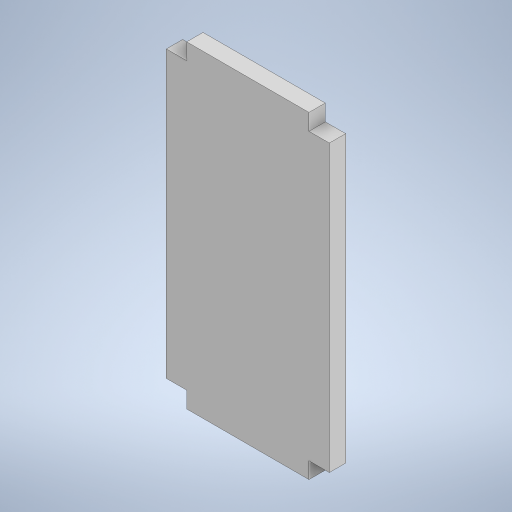
# Autodesk Inventor part: Tussen30_AUG
Saved by Autodesk Inventor 2023.4 (Build 274418000, 418)
## iProperties
Created: 2024-07-29
Part Number: Tussen30_AUG
Material: Generic
Document SubType Name: Modeling
Designer: cthey
Density: 1 g/cm^3
Appearance: Default
Author: cthey
Autodesk Inventor part; units mm, degrees
ref_plane "YZ Plane" through (0, 0, 0) normal (1, 0, 0) x (0, 1, 0)
ref_plane "XZ Plane" through (0, 0, 0) normal (0, 1, 0) x (-1, 0, 0)
ref_plane "XY Plane" through (0, 0, 0) normal (0, 0, 1) x (1, 0, 0)
sketch "Sketch1" plane through (0, 0, 0) normal (0, 0, 1) x (1, 0, 0)
  line L0 (0, 0) -> (30, 0)
  line L1 (30, 0) -> (30, 78)
  line L2 (30, 78) -> (0, 78)
  line L3 (0, 78) -> (0, 0)
  line L4 (-5, 74) -> (35, 74)
  line L5 (35, 74) -> (35, 4)
  line L6 (35, 4) -> (-5, 4)
  line L7 (-5, 4) -> (-5, 74)
  point P0 (0, 4)
  point P1 (30, 4)
  point P2 (30, 74)
  point P3 (0, 74)
  dimension "d0" = 78
  dimension "d1" = 30
  dimension "d2" = 40
  dimension "d3" = 5
  dimension "d4" = 4
  dimension "d5" = 4
  constraints: 16 end point, 4 parallel, 2 horizontal, 2 perpendicular
  measures "d0" distance between parallel lines of L0 L2
  measures "d1" distance between parallel lines of L1 L3
  measures "d2" distance between parallel lines of L5 L7
  measures "d3" distance between parallel lines of L3 L7
  measures "d4" distance between parallel lines of L0 L6
  measures "d5" distance between parallel lines of L2 L4
extrude "Extrusion1" add sketch "Sketch1" along normal blind 4
body "Solid1"
